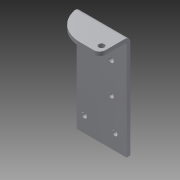
# Autodesk Inventor part: Pneumatic Piston Front Flange (Right Custom)
Saved by Autodesk Inventor 2014 (Build 180170000, 170)
## iProperties
Created: 2014-01-17
Part Number: Pneumatic Piston Front Flange (Right Custom)
Material: Aluminum 6061
Document SubType Name: Sheet Metal
Designer: Michael
Density: 2.71 g/cm^3
Sheet Metal Rule: Default
Appearance: Aluminum - Flat
Flat Pattern Width: 13.1491 cm
Flat Pattern Length: 4.1275 cm
Flat Pattern Area: 54.273 cm^2
Sheet Metal Width: 5.177 in
Sheet Metal Length: 1.625 in
Sheet Metal Area: 8.412 in^2
Author: Michael
Autodesk Inventor part; units mm, degrees
ref_plane "YZ Plane" through (0, 0, 0) normal (1, 0, 0) x (0, 1, 0)
ref_plane "XZ Plane" through (0, 0, 0) normal (0, 1, 0) x (-1, 0, 0)
ref_plane "XY Plane" through (0, 0, 0) normal (0, 0, 1) x (1, 0, 0)
sketch "Sketch1" plane through (0, 0, 0) normal (0, 0, 1) x (1, 0, 0)
  line L0 (0, 0) -> (41.275, 0)
  line L1 (41.275, 0) -> (41.275, 106.3625)
  line L2 (41.275, 106.3625) -> (0, 106.3625)
  line L3 (0, 106.3625) -> (0, 0)
  circle A0 centre (6.35, 12.7) radius 2.0701
  line L4 (0, 12.7) -> (41.275, 12.7) construction
  circle A1 centre (31.75, 12.7) radius 2.0701
  circle A2 centre (28.575, 38.1) radius 2.0701
  circle A3 centre (28.575, 63.5) radius 2.0701
  circle A4 centre (28.575, 88.9) radius 2.0701
  dimension "d0" = 41.275
  dimension "d1" = 106.3625
  dimension "d2" = 4.1402
  dimension "d3" = 6.35
  dimension "d6" = 25.4
  dimension "d22" = 12.7
  dimension "d36" = 12.7
  dimension "d37" = 38.1
  dimension "d40" = 25.4
  measures "d0" distance of L2.end L1.end
  measures "d1" distance of L1.end L0.end
  measures "d2" diameter of A0
  measures "d3" distance from line of L3 A0.centre
  measures "d6" distance of A0.centre A1.centre
  measures "d22" distance between parallel lines of L0 L4
  measures "d36" distance from line of L1 A2.centre
  measures "d37" distance from line of L0 A2.centre
  measures "d40" distance of A2.centre A3.centre
extrude "Plate1" add sketch "Sketch1" along normal blind 3.175
sketch "Sketch2" plane through (0, 107.6325, 4.445) normal (0, 1, 0) x (-1, 0, 0)
  line L0 (-41.275, 0) -> (0, 0)
  line L1 (0, 0) -> (0, 20.955)
  line L2 (0, 20.955) -> (-41.275, 20.955)
  line L3 (-41.275, 20.955) -> (-41.275, 0)
  constraints: 6 end point, 1 horizontal, 1 perpendicular, 1 vertical
edge flange "Flange1" height 25.4 angle 90 thickness 3.175 bend radius 1.27 thickness toward (0, 1, 0) relief straight relief width 3.175 relief depth 1.5875 edges at (20.6375, 106.3625, 3.175) wall of the first edge with corners at (41.275, 107.6325, 4.445) (0, 107.6325, 4.445) (0, 107.6325, 25.4) (41.275, 107.6325, 25.4)
bend "Bend1"
corner "Corner1"
sketch "Sketch4" plane through (0, 110.8075, 25.4) normal (0, 1, 0) x (1, 0, 0)
  line L0 (41.275, 0) -> (0, 0) projected
  line L1 (41.275, 20.955) -> (41.275, 0) projected
  circle A0 centre (22.225, 6.35) radius 2.3749
  line L2 (0, 20.955) -> (41.275, 20.955)
  line L3 (41.275, 20.955) -> (41.275, 22.225)
  line L4 (19.05, 0) -> (20.1397, 0)
  line L5 (0, 0) -> (0, 20.955)
  line L6 (19.05, 0) -> (19.05, 0)
  line L7 (41.275, 0) -> (41.275, 22.225)
  line L8 (41.275, 20.955) -> (0, 20.955) projected
  line L9 (0, 0) -> (0, 20.955) projected
  line L10 (0, 17.78) -> (13.0346, 3.1812)
  line L11 (28.575, 9.525) -> (28.575, 20.955)
  arc A1 (13.0346, 3.1812) -> (19.5948, 0.0156) centre (20.1397, 9.525) ccw
  arc A2 (19.5948, 0.0156) -> (28.575, 9.525) centre (19.05, 9.525) ccw
  line L12 (0, 17.78) -> (0, 20.955)
  line L13 (0, 20.955) -> (28.575, 20.955)
  line L14 (28.575, 20.955) -> (28.575, 9.525)
  line L15 (28.575, 20.955) -> (0, 20.955)
  line L16 (0, 20.955) -> (0, 17.78)
  line L17 (0, 17.78) -> (13.0346, 3.1812)
  point P0 (0, 25.4)
  point P1 (15.875, 0)
  dimension "d28" = 4.7498
  dimension "d29" = 6.35
  dimension "d30" = 19.05
  dimension "d45" = 3.175
  dimension "d46" = 6.35
  dimension "d47" = 6.35
  dimension "d48" = 9.525
  constraints: 28 end point, 8 point on line, 6 collinear, 6 tangent, 4 point on circle, 3 centre point, 3 perpendicular, 2 parallel, 1 equal radius, 1 horizontal
  measures "d28" diameter of A0
  measures "d29" distance from line of L0 A0.centre
  measures "d30" distance from line of L1 A0.centre
  measures "d45" distance from line of L10.start L2
  measures "d46" distance from line of A0.centre L11
  measures "d47" horizontal distance of A0.centre point (15.875, 0)
  measures "d48" radius of A1
extrude "Cut2" cut sketch "Sketch4" against normal blind 3.175 contours L0 L5 L10 A1 A2 L11 L2 L1 | A0
fillet "Fillet3" radius 6.35 2 edges at (0, 109.22, 7.62) (28.575, 109.22, 4.445)
equation "\"d31\" = Thickness"
equation "\"d12\" = BendReliefWidth"
equation "\"d13\" = BendReliefDepth"
equation "\"d14\" = MinimumRemnant"
equation "\"d15\" = BendRadius"
equation "\"d19\" = CornerReliefSize"
equation "\"d20\" = GapSize"
equation "\"d21\" = JacobiRadiusSize"
equation "\"BendRadius\" = Thickness"
equation "\"BendReliefWidth\" = Thickness"
equation "\"BendReliefDepth\" = 0.5 * Thickness"
equation "\"CornerReliefSize\" = 4 * Thickness"
equation "\"MinimumRemnant\" = 2 * Thickness"
equation "\"TransitionRadius\" = BendRadius"
equation "\"JacobiRadiusSize\" = BendRadius"
equation "\"GapSize\" = Thickness"
equation "\"d11\" = BendRadius"
equation "\"Thickness\" = 3.175"
body "Solid1"
